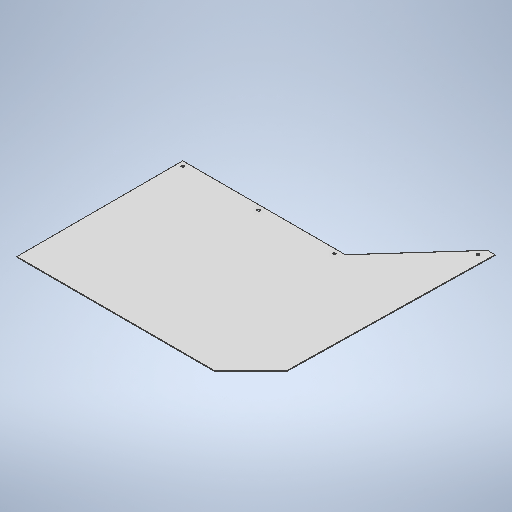
# Autodesk Inventor part: BSH 015 board cone wall
Saved by Autodesk Inventor 2025 (Build 290162010, 162A)
## iProperties
Created: 2024-07-23
Part Number: BSH 015 board cone wall
Material: 09g2s
Document SubType Name: Sheet Metal
Designer: admin
Mass: 17038.2 g
Surface Area: 14581.9 cm^2
Volume: 2170.48 cm^3
Density: 7.85 g/cm^3
Sheet Metal Rule: AISI304 3mm Die 32
Sheet Metal Width: 996,593 mm
Sheet Metal Length: 1034,076 mm
Sheet Metal Area: 1030552,820 mm^2
Appearance: Default
Flat Pattern Width: 99.6593 cm
Flat Pattern Length: 103.408 cm
Flat Pattern Area: 10305.5 cm^2
Stock Number: БШК 015 борт конус стенка
Author: admin
Autodesk Inventor part; units mm, degrees
ref_plane "YZ Plane" through (0, 0, 0) normal (1, 0, 0) x (0, 1, 0)
ref_plane "XZ Plane" through (0, 0, 0) normal (0, 1, 0) x (-1, 0, 0)
ref_plane "XY Plane" through (0, 0, 0) normal (0, 0, 1) x (1, 0, 0)
sketch "Sketch8" plane through (0, 0, 0) normal (0, 0, 1) x (1, 0, 0)
  line L0 (0, 2897) -> (1200, 2897)
  line L1 (1200, 2897) -> (1200, 0)
  line L2 (1200, 0) -> (0, 0)
  line L3 (0, 0) -> (0, 2897)
  line L4 (0, 2897) -> (1200, 0) construction
  line L5 (1200, 2897) -> (0, 0) construction
  line L6 (947, 0) -> (1097, 150)
  line L7 (1097, 150) -> (1147, 2897)
  line L8 (0, 700) -> (1200, 700)
  line L9 (1112.5806, 1006) -> (837.057, 700)
  line L10 (110.253, 0) -> (110.253, 700)
  line L11 (796.688, 700) -> (1081.2157, 1016)
  line L12 (1081.2157, 1016) -> (1112.7627, 1016)
  point P0 (600, 1448.5)
  point P1 (1107.0109, 700)
  dimension "d43" = 1200
  dimension "d44" = 2897
  dimension "d45" = 53
  dimension "d46" = 947
  dimension "d47" = 150
  dimension "d48" = 103
  dimension "d49" = 700
  dimension "d55" = 306
  dimension "d57" = 110.253
  dimension "d61" = 48
  dimension "d65" = 10
  dimension "d66" = 30
  measures "d43" distance of L1.end L2.end
  measures "d44" distance of L0.end L1.end
  measures "d45" distance of L0.end L7.end
  measures "d46" distance of point (0, 0) L6.start
  measures "d47" distance from line of L2 L6.end
  measures "d48" distance from line of L1 L6.end
  measures "d49" distance of L1.end L8.end
  measures "d55" distance from line of L8 L9.start
  measures "d57" distance between parallel lines of L3 L10
  measures "d61" angle of L8 L9
  measures "d65" vertical distance of L9.start L12.end
  measures "d66" distance between parallel lines of L9 L11
extrude "Plate4" add sketch "Sketch8" against normal blind 3 contours L7 L9 L8 L11 L12 | L8 L7 L6 L2 L10 | L7 L8 L9
chamfer "Corner Chamfer1" distance 6 angle 45 2 edges at (947, 0, -1.5) (1097, 150, -1.5)
sketch "Sketch9" plane through (0, 0, 0) normal (0, 0, 1) x (1, 0, 0)
  line L0 (1097.1092, 155.999) -> (1092.7574, 145.7574) projected
  line L1 (1097.1092, 155.999) -> (1112.7627, 1016) projected
  line L2 (1112.7627, 1016) -> (1081.2157, 1016) projected
  line L3 (1081.2157, 1016) -> (796.688, 700) projected
  line L4 (796.688, 700) -> (110.253, 700) projected
  line L5 (110.253, 700) -> (110.253, 0) projected
  line L6 (110.253, 0) -> (941, 0) projected
  line L7 (951.2426, 4.2426) -> (941, 0) projected
  line L8 (951.2426, 4.2426) -> (1092.7574, 145.7574) projected
  circle A0 centre (130.253, 680) radius 5.5
  point P0 (0, 0)
  dimension "d67" = 11
  dimension "d68" = 20
  dimension "d69" = 20
  constraints: 1 centre point
  measures "d67" diameter of A0
  measures "d68" distance from line of L4 A0.centre
  measures "d69" distance from line of L5 A0.centre
extrude "Extrusion2" cut sketch "Sketch9" against normal through all contours A0
pattern_linear "Rectangular Pattern2" count 3 spacing 320 along (1, 0, 0) of "Extrusion2"
sketch "Sketch10" plane through (0, 0, 0) normal (0, 0, 1) x (1, 0, 0)
  circle A0 centre (770.253, 680) radius 5.5 projected
  circle A1 centre (450.253, 680) radius 5.5 projected
  circle A2 centre (130.253, 680) radius 5.5 projected
  line L0 (1097.1092, 155.999) -> (1092.7574, 145.7574) projected
  line L1 (1097.1092, 155.999) -> (1112.7627, 1016) projected
  line L2 (1112.7627, 1016) -> (1081.2157, 1016) projected
  line L3 (1081.2157, 1016) -> (796.688, 700) projected
  line L4 (796.688, 700) -> (110.253, 700) projected
  line L5 (110.253, 700) -> (110.253, 0) projected
  line L6 (110.253, 0) -> (941, 0) projected
  line L7 (951.2426, 4.2426) -> (941, 0) projected
  line L8 (951.2426, 4.2426) -> (1092.7574, 145.7574) projected
  circle A3 centre (1076.0047, 980.323) radius 5.5
  line L9 (1081.2157, 1016) -> (1112.254, 988.053)
  line L10 (1097.1092, 155.999) -> (1112.7627, 1016) projected
  point P0 (0, 0)
  dimension "d75" = 20
  dimension "d76" = 30
  constraints: 2 end point, 1 centre point, 1 equal radius, 1 perpendicular, 1 point on line
  measures "d75" distance from line of A3.centre L3
  measures "d76" distance from line of L9 A3.centre
extrude "Extrusion3" cut sketch "Sketch10" against normal through all contours A3
equation "\"d50\" = Thickness"
equation "\"BendReliefWidth\" = Thickness"
equation "\"BendReliefDepth\" = 0.5 * Thickness"
equation "\"CornerReliefSize\" = 4 * Thickness"
equation "\"MinimumRemnant\" = 2 * Thickness"
equation "\"TransitionRadius\" = BendRadius"
equation "\"JacobiRadiusSize\" = BendRadius"
equation "\"GapSize\" = Thickness"
equation "\"Thickness\" = 3"
equation "\"BendRadius\" = 5"
body "Solid2"
